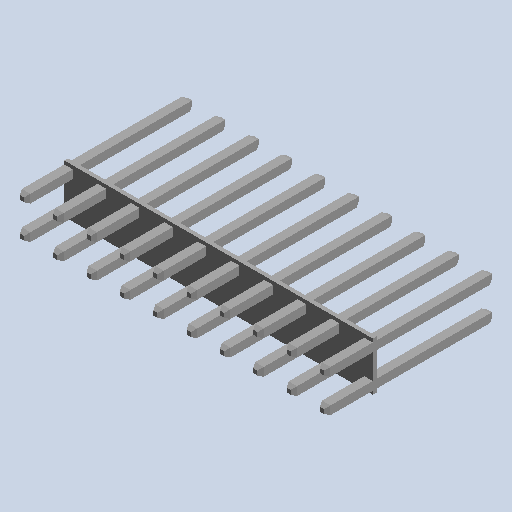
# Autodesk Inventor part: P3TW-10-11-T-D-250-080
Saved by Autodesk Inventor 2024.2 (Build 282272000, 272)
## iProperties
Category: PARTsolutions
Company: SAMTEC
Part Number: P3TW-10-11-T-D-250-080
Material: Generic
Catalog Web Link: www.cadenas.de
Description: TW-TH Pin-TW-TH Series
Vendor: SAMTEC
Document SubType Name: Modeling
Designer: partserver
Manufacturer: SAMTEC
Mass: 0.0621315 g
Surface Area: 5.07361 cm^2
Volume: 0.0621315 cm^3
Density: 1 g/cm^3
Appearance: PSOLRGB-191-191-191
PSOL_IDENT_0: {$CADENAS_DATA\23d-libs\samtec\modelling\tw\parts\tw-th_pin.prj},243 {VTYP=3D},{NB=P3TW-10-11-T-D-25
PSOL_IDENT_1: 0-080},{LINA=P3TW-10-11-T-D-250-080},{NN=TW-TH Pin},{DATE=29.08.2019 09:17:22},{GEOMDATE=10.06.2019
PSOL_IDENT_2: 09:23:15},{VERSION=},{LINEID=10},{WBVAR=PINS,LEADST,PLOPT,ROWOPT,STACKERH,TAILL,POLARIZE},{WBNUMERIC=
PSOL_IDENT_3: STACKERH}  {NB=P3TW-10-11-T-D-250-080},{LINA=P3TW-10-11-T-D-250-080},{KT=DUMMY},{PN=TW-10-11-T-D-250
PSOL_IDENT_4: -080},{SERIES=TW-TH},{PINS=10},{LEADST=11},{LEADSTALG=},{PLOPT=T},{PLOPTALG= '-L','10micro\" (0,25 m
PSOL_IDENT_5: icrom) Gold on contact, Matte Tin on tail','-S','30micro\" (0,76 microm) Gold on contact, Matte Tin
PSOL_IDENT_6: on tail' },{ROWOPT=D},{ROWOPTALG= '5','5:Five Row','6','6:Six Row','D','D:Double Row','Q','Q:Quad Ro
PSOL_IDENT_7: w','S','S:Single row','T','T:Triple Row' },{STACKERH=250},{STACKERHALG=[120:397/5]},{TAILL=080},{TAI
PSOL_IDENT_8: LLALG='000','005','010','015','020','025','030','035','040','045','050','055','060','065','070','075'
PSOL_IDENT_9: ,'080','085','090','095','100','105','110','115','120','125','130','135','140','145'},{ALIGNMENTALG=
PSOL_IDENT_10: x},{POLARIZE=Not Selected},{POLARIZEALG='001','002','003','004','005','006','007','008','009','010','
PSOL_IDENT_11: 011','012','013','014','015','016','017','018','019','020'},{POLARIZEPN=},{KOPTALG= '','Not Selected'
PSOL_IDENT_12: ,'-P','P:Plastic Pick and Place Pad' },{TROPTALG= '','Not Selected','-TR','TR:Tape and Reel' },{IMAT=
PSOL_IDENT_13: Black Liquid Crystal Polymer},{TM=Phosphor Bronze},{PLAT=Au or Sn over 50micro\" (1,27 microm) Ni},{
PSOL_IDENT_14: CR=5.2 A per pin (1 pin powered per row)},{OTEMP=-55°C to +125°C},{ROHSC=Yes},{L=0.7874},{W=0.1574},
PSOL_IDENT_15: {OAL=0.397},{STACKERHMAX=397},{POLMAX='001','002','003','004','005','006','007','008','009','010','0
PSOL_IDENT_16: 11','012','013','014','015','016','017','018','019','020','021','022','023','024','025','026','027','
PSOL_IDENT_17: 028','029','030','031','032','033','034','035','036','037','038','039','040','041','042','043','044'
PSOL_IDENT_18: ,'045','046','047','048','049','050','051','052','053','054','055','056','057','058','059','060','06
PSOL_IDENT_19: 1','062','063','064','065','066','067','068','069','070','071','072','073','074','075','076','077','
PSOL_IDENT_20: 078','079','080','081','082','083','084','085','086','087','088','089','090','091','092','093','094'
PSOL_IDENT_21: ,'095','096','097','098','099','100','101','102','103','104','105','106','107','108','109','110','11
PSOL_IDENT_22: 1','112','113','114','115','116','117','118','119','120','121','122','123','124','125','126','127','
PSOL_IDENT_23: 128','129','130','131','132','133','134','135','136','137','138','139','140','141','142','143','144'
PSOL_IDENT_24: ,'145','146','147','148','149','150','151','152','153','154','155','156','157','158','159','160','16
PSOL_IDENT_25: 1','162','163','164','165','166','167','168','169','170','171','172','173','174','175','176','177','
PSOL_IDENT_26: 178','179','180','181','182','183','184','185','186','187','188','189','190','191','192','193','194'
PSOL_IDENT_27: ,'195','196','197','198','199','200','201','202','203','204','205','206','207','208','209','210','21
PSOL_IDENT_28: 1','212','213','214','215','216','217','218','219','220','221','222','223','224','225','226','227','
PSOL_IDENT_29: 228','229','230','231','232','233','234','235','236','237','238','239','240','241','242','243','244'
PSOL_IDENT_30: ,'245','246','247','248','249','250','251','252','253','254','255','256','257','258','259','260','26
PSOL_IDENT_31: 1','262','263','264','265','266','267','268','269','270','271','272','273','274','275','276','277','
PSOL_IDENT_32: 278','279','280','281','282','283','284','285','286','287','288','289','290','291','292','293','294'
PSOL_IDENT_33: ,'295','296','297','298','299','300'},{TEST2='001','002','003','004','005','006','007','008','009','
PSOL_IDENT_34: 010','011','012','013','014','015','016','017','018','019','020'},{TRUNC=20},{MIN=0.147},{PINSNUM=10
PSOL_IDENT_35: },{POLLR=0},{TAILLMAX=147},{TAILLRANGE='000','005','010','015','020','025','030','035','040','045','
PSOL_IDENT_36: 050','055','060','065','070','075','080','085','090','095','100','105','110','115','120','125','130'
PSOL_IDENT_37: ,'135','140','145','150','155','160','165','170','175','180','185','190','195','200','205','210','21
PSOL_IDENT_38: 5','220','225','230','235','240','245','250','255','260','265','270','275','280','285','290','295','
PSOL_IDENT_39: 300','305','310','315','320','325','330','335','340','345','350','355','360','365','370','375','380'
PSOL_IDENT_40: ,'385','390','395','400','405','410','415','420','425','430','435','440','445','450','455','460','46
PSOL_IDENT_41: 5','470','475','480','485','490','495','500','505','510','515','520','525','530','535','540','545','
PSOL_IDENT_42: 550','555','560','565','570','575','580','585','590','595','600','605','610','615','620','625','630'
PSOL_IDENT_43: ,'635','640','645','650','655','660','665','670','675','680','685','690','695','700','705','710','71
PSOL_IDENT_44: 5','720','725','730','735','740','745','750','755','760','765','770','775','780','785','790','795','
PSOL_IDENT_45: 800','805','810','815','820','825','830','835','840','845','850','855','860','865','870','875','880'
PSOL_IDENT_46: ,'885','890','895','900','905','910','915','920','925','930','935','940','945','950','955','960','96
PSOL_IDENT_47: 5','970','975','980','985','990','995'},{TAILLTRUNC=30},{TAILLNUM=0.08},{ROWNO=2},{POLPLANEPOS=0},{P
PSOL_IDENT_48: OLPINPOS=0},{COLOR=0.75,0.75,0.75,0.00}
NB: P3TW-10-11-T-D-250-080
NN: TW-TH Pin
NT: TW-TH Series
NBSYN: P3$PN.
LINA: P3TW-10-11-T-D-250-080
CATALOG: Samtec
SERIES: TW-TH
PINS: 10
LEADST: 11
PLOPT: -T: Matte Tin Contact and Tail
ROWOPT: D:Double Row
STACKERH: 250
TAILL: 080
POLARIZE: Not Selected
IMAT: Black Liquid Crystal Polymer
TM: Phosphor Bronze
PLAT: Au or Sn over 50micro" (1,27 microm) Ni
CR: 5.2 A per pin (1 pin powered per row)
OTEMP: -55°C to +125°C
ROHSC: Yes
POLMAX: '001','002','003','004','005','006','007','008','009','010','011','012','013','014','015','016','017','018','019','020','021','022','023','024','025','026','027','028','029','030','031','032','033','034','035','036','037','038','039','040','041','042','043','044','045','046','047','048','049','050','051','052','053','054','055','056','057','058','059','060','061','062','063','064','065','066','067','068','069','070','071','072','073','074','075','076','077','078','079','080','081','082','083','084','085','086','087','088','089','090','091','092','093','094','095','096','097','098','099','100','101','102','103','104','105','106','107','108','109','110','111','112','113','114','115','116','117','118','119','120','121','122','123','124','125','126','127','128','129','130','131','132','133','134','135','136','137','138','139','140','141','142','143','144','145','146','147','148','149','150','151','152','153','154','155','156','157','158','159','160','161','162','163','164','165','166','167','168','169','170','171','172','173','174','175','176','177','178','179','180','181','182','183','184','185','186','187','188','189','190','191','192','193','194','195','196','197','198','199','200','201','202','203','204','205','206','207','208','209','210','211','212','213','214','215','216','217','218','219','220','221','222','223','224','225','226','227','228','229','230','231','232','233','234','235','236','237','238','239','240','241','242','243','244','245','246','247','248','249','250','251','252','253','254','255','256','257','258','259','260','261','262','263','264','265','266','267','268','269','270','271','272','273','274','275','276','277','278','279','280','281','282','283','284','285','286','287','288','289','290','291','292','293','294','295','296','297','298','299','300'
TAILLRANGE: '000','005','010','015','020','025','030','035','040','045','050','055','060','065','070','075','080','085','090','095','100','105','110','115','120','125','130','135','140','145','150','155','160','165','170','175','180','185','190','195','200','205','210','215','220','225','230','235','240','245','250','255','260','265','270','275','280','285','290','295','300','305','310','315','320','325','330','335','340','345','350','355','360','365','370','375','380','385','390','395','400','405','410','415','420','425','430','435','440','445','450','455','460','465','470','475','480','485','490','495','500','505','510','515','520','525','530','535','540','545','550','555','560','565','570','575','580','585','590','595','600','605','610','615','620','625','630','635','640','645','650','655','660','665','670','675','680','685','690','695','700','705','710','715','720','725','730','735','740','745','750','755','760','765','770','775','780','785','790','795','800','805','810','815','820','825','830','835','840','845','850','855','860','865','870','875','880','885','890','895','900','905','910','915','920','925','930','935','940','945','950','955','960','965','970','975','980','985','990','995'
SUPPLIER: SAMTEC
ARTICLENO: P3TW-10-11-T-D-250-080
BOMINFO: P3TW-10-11-T-D-250-080
CREATOR: CADENAS GmbH
Title: P3TW-10-11-T-D-250-080
Author: Cadenas PARTsolutions
Comments: TW-TH Series
Autodesk Inventor part; units mm, degrees
sketch "Sketch_2" plane through (9.254, 0, 0) normal (1, 0, 0) x (0, 0, -1)
  line L0 (-1.4605, 0.762) -> (-1.254, 0.762)
  line L1 (-1.254, 0.762) -> (-1.254, -1.778)
  line L2 (-1.254, -1.778) -> (-1.127, -2.032)
  line L3 (-1.127, -2.032) -> (-0.873, -2.032)
  line L4 (-0.873, -2.032) -> (-0.746, -1.778)
  line L5 (-0.746, -1.778) -> (-0.746, 0.762)
  line L6 (-0.746, 0.762) -> (0.746, 0.762)
  line L7 (0.746, 0.762) -> (0.746, -1.778)
  line L8 (0.746, -1.778) -> (0.873, -2.032)
  line L9 (0.873, -2.032) -> (1.127, -2.032)
  line L10 (1.127, -2.032) -> (1.254, -1.778)
  line L11 (1.254, -1.778) -> (1.254, 0.762)
  line L12 (1.254, 0.762) -> (1.4605, 0.762)
  line L13 (1.4605, 0.762) -> (1.4605, 0.9906)
  line L14 (1.4605, 0.9906) -> (1.254, 0.9906)
  line L15 (1.254, 0.9906) -> (1.254, 7.7978)
  line L16 (1.254, 7.7978) -> (1.127, 8.0518)
  line L17 (1.127, 8.0518) -> (0.873, 8.0518)
  line L18 (0.873, 8.0518) -> (0.746, 7.7978)
  line L19 (0.746, 7.7978) -> (0.746, 0.9906)
  line L20 (0.746, 0.9906) -> (-0.746, 0.9906)
  line L21 (-0.746, 0.9906) -> (-0.746, 7.7978)
  line L22 (-0.746, 7.7978) -> (-0.873, 8.0518)
  line L23 (-0.873, 8.0518) -> (-1.127, 8.0518)
  line L24 (-1.127, 8.0518) -> (-1.254, 7.7978)
  line L25 (-1.254, 7.7978) -> (-1.254, 0.9906)
  line L26 (-1.254, 0.9906) -> (-1.4605, 0.9906)
  line L27 (-1.4605, 0.9906) -> (-1.4605, 0.762)
  constraints: 56 end point
extrude "Extrusion1" add sketch "Sketch_2" against normal blind 18.508
sketch "Sketch_1" plane through (0, 0, 0) normal (0, 0, 1) x (1, 0, 0)
  line L0 (-109.4334, 38.1) -> (-109.4334, -38.1)
  line L1 (-109.4334, -38.1) -> (56.7986, -38.1)
  line L2 (56.7986, -38.1) -> (56.7986, 38.1)
  line L3 (56.7986, 38.1) -> (-109.4334, 38.1)
  line L4 (-93.4603, 0.762) -> (-93.2538, 0.762)
  line L5 (-93.2538, 0.762) -> (-93.2538, -1.778)
  line L6 (-93.2538, -1.778) -> (-93.1268, -2.032)
  line L7 (-93.1268, -2.032) -> (-92.8728, -2.032)
  line L8 (-92.8728, -2.032) -> (-92.7458, -1.778)
  line L9 (-92.7458, -1.778) -> (-92.7458, 0.762)
  line L10 (-92.7458, 0.762) -> (-91.2538, 0.762)
  line L11 (-91.2538, 0.762) -> (-91.2538, -1.778)
  line L12 (-91.2538, -1.778) -> (-91.1268, -2.032)
  line L13 (-91.1268, -2.032) -> (-90.8728, -2.032)
  line L14 (-90.8728, -2.032) -> (-90.7458, -1.778)
  line L15 (-90.7458, -1.778) -> (-90.7458, 0.762)
  line L16 (-90.7458, 0.762) -> (-89.2538, 0.762)
  line L17 (-89.2538, 0.762) -> (-89.2538, -1.778)
  line L18 (-89.2538, -1.778) -> (-89.1268, -2.032)
  line L19 (-89.1268, -2.032) -> (-88.8728, -2.032)
  line L20 (-88.8728, -2.032) -> (-88.7458, -1.778)
  line L21 (-88.7458, -1.778) -> (-88.7458, 0.762)
  line L22 (-88.7458, 0.762) -> (-87.2538, 0.762)
  line L23 (-87.2538, 0.762) -> (-87.2538, -1.778)
  line L24 (-87.2538, -1.778) -> (-87.1268, -2.032)
  line L25 (-87.1268, -2.032) -> (-86.8728, -2.032)
  line L26 (-86.8728, -2.032) -> (-86.7458, -1.778)
  line L27 (-86.7458, -1.778) -> (-86.7458, 0.762)
  line L28 (-86.7458, 0.762) -> (-85.2538, 0.762)
  line L29 (-85.2538, 0.762) -> (-85.2538, -1.778)
  line L30 (-85.2538, -1.778) -> (-85.1268, -2.032)
  line L31 (-85.1268, -2.032) -> (-84.8728, -2.032)
  line L32 (-84.8728, -2.032) -> (-84.7458, -1.778)
  line L33 (-84.7458, -1.778) -> (-84.7458, 0.762)
  line L34 (-84.7458, 0.762) -> (-83.2538, 0.762)
  line L35 (-83.2538, 0.762) -> (-83.2538, -1.778)
  line L36 (-83.2538, -1.778) -> (-83.1268, -2.032)
  line L37 (-83.1268, -2.032) -> (-82.8728, -2.032)
  line L38 (-82.8728, -2.032) -> (-82.7458, -1.778)
  line L39 (-82.7458, -1.778) -> (-82.7458, 0.762)
  line L40 (-82.7458, 0.762) -> (-81.2538, 0.762)
  line L41 (-81.2538, 0.762) -> (-81.2538, -1.778)
  line L42 (-81.2538, -1.778) -> (-81.1268, -2.032)
  line L43 (-81.1268, -2.032) -> (-80.8728, -2.032)
  line L44 (-80.8728, -2.032) -> (-80.7458, -1.778)
  line L45 (-80.7458, -1.778) -> (-80.7458, 0.762)
  line L46 (-80.7458, 0.762) -> (-79.2538, 0.762)
  line L47 (-79.2538, 0.762) -> (-79.2538, -1.778)
  line L48 (-79.2538, -1.778) -> (-79.1268, -2.032)
  line L49 (-79.1268, -2.032) -> (-78.8728, -2.032)
  line L50 (-78.8728, -2.032) -> (-78.7458, -1.778)
  line L51 (-78.7458, -1.778) -> (-78.7458, 0.762)
  line L52 (-78.7458, 0.762) -> (-77.2538, 0.762)
  line L53 (-77.2538, 0.762) -> (-77.2538, -1.778)
  line L54 (-77.2538, -1.778) -> (-77.1268, -2.032)
  line L55 (-77.1268, -2.032) -> (-76.8728, -2.032)
  line L56 (-76.8728, -2.032) -> (-76.7458, -1.778)
  line L57 (-76.7458, -1.778) -> (-76.7458, 0.762)
  line L58 (-76.7458, 0.762) -> (-75.2539, 0.762)
  line L59 (-75.2539, 0.762) -> (-75.2539, -1.778)
  line L60 (-75.2539, -1.778) -> (-75.1268, -2.032)
  line L61 (-75.1268, -2.032) -> (-74.8728, -2.032)
  line L62 (-74.8728, -2.032) -> (-74.7459, -1.778)
  line L63 (-74.7459, -1.778) -> (-74.7459, 0.762)
  line L64 (-74.7459, 0.762) -> (-73.2539, 0.762)
  line L65 (-73.2539, 0.762) -> (-73.2539, -1.778)
  line L66 (-73.2539, -1.778) -> (-73.1269, -2.032)
  line L67 (-73.1269, -2.032) -> (-72.8729, -2.032)
  line L68 (-72.8729, -2.032) -> (-72.7459, -1.778)
  line L69 (-72.7459, -1.778) -> (-72.7459, 0.762)
  line L70 (-72.7459, 0.762) -> (-71.2539, 0.762)
  line L71 (-71.2539, 0.762) -> (-71.2539, -1.778)
  line L72 (-71.2539, -1.778) -> (-71.1269, -2.032)
  line L73 (-71.1269, -2.032) -> (-70.8729, -2.032)
  line L74 (-70.8729, -2.032) -> (-70.7459, -1.778)
  line L75 (-70.7459, -1.778) -> (-70.7459, 0.762)
  line L76 (-70.7459, 0.762) -> (-69.2539, 0.762)
  line L77 (-69.2539, 0.762) -> (-69.2539, -1.778)
  line L78 (-69.2539, -1.778) -> (-69.1269, -2.032)
  line L79 (-69.1269, -2.032) -> (-68.8729, -2.032)
  line L80 (-68.8729, -2.032) -> (-68.7459, -1.778)
  line L81 (-68.7459, -1.778) -> (-68.7459, 0.762)
  line L82 (-68.7459, 0.762) -> (-67.2539, 0.762)
  line L83 (-67.2539, 0.762) -> (-67.2539, -1.778)
  line L84 (-67.2539, -1.778) -> (-67.1269, -2.032)
  line L85 (-67.1269, -2.032) -> (-66.8729, -2.032)
  line L86 (-66.8729, -2.032) -> (-66.7459, -1.778)
  line L87 (-66.7459, -1.778) -> (-66.7459, 0.762)
  line L88 (-66.7459, 0.762) -> (-65.2539, 0.762)
  line L89 (-65.2539, 0.762) -> (-65.2539, -1.778)
  line L90 (-65.2539, -1.778) -> (-65.1269, -2.032)
  line L91 (-65.1269, -2.032) -> (-64.8729, -2.032)
  line L92 (-64.8729, -2.032) -> (-64.7459, -1.778)
  line L93 (-64.7459, -1.778) -> (-64.7459, 0.762)
  line L94 (-64.7459, 0.762) -> (-63.2539, 0.762)
  line L95 (-63.2539, 0.762) -> (-63.2539, -1.778)
  line L96 (-63.2539, -1.778) -> (-63.1269, -2.032)
  line L97 (-63.1269, -2.032) -> (-62.8729, -2.032)
  line L98 (-62.8729, -2.032) -> (-62.7459, -1.778)
  line L99 (-62.7459, -1.778) -> (-62.7459, 0.762)
  line L100 (-62.7459, 0.762) -> (-61.2539, 0.762)
  line L101 (-61.2539, 0.762) -> (-61.2539, -1.778)
  line L102 (-61.2539, -1.778) -> (-61.1269, -2.032)
  line L103 (-61.1269, -2.032) -> (-60.8729, -2.032)
  line L104 (-60.8729, -2.032) -> (-60.7459, -1.778)
  line L105 (-60.7459, -1.778) -> (-60.7459, 0.762)
  line L106 (-60.7459, 0.762) -> (-59.2539, 0.762)
  line L107 (-59.2539, 0.762) -> (-59.2539, -1.778)
  line L108 (-59.2539, -1.778) -> (-59.1269, -2.032)
  line L109 (-59.1269, -2.032) -> (-58.8729, -2.032)
  line L110 (-58.8729, -2.032) -> (-58.7459, -1.778)
  line L111 (-58.7459, -1.778) -> (-58.7459, 0.762)
  line L112 (-58.7459, 0.762) -> (-57.2539, 0.762)
  line L113 (-57.2539, 0.762) -> (-57.2539, -1.778)
  line L114 (-57.2539, -1.778) -> (-57.1269, -2.032)
  line L115 (-57.1269, -2.032) -> (-56.8729, -2.032)
  line L116 (-56.8729, -2.032) -> (-56.7459, -1.778)
  line L117 (-56.7459, -1.778) -> (-56.7459, 0.762)
  line L118 (-56.7459, 0.762) -> (-55.2539, 0.762)
  line L119 (-55.2539, 0.762) -> (-55.2539, -1.778)
  line L120 (-55.2539, -1.778) -> (-55.1269, -2.032)
  line L121 (-55.1269, -2.032) -> (-54.8729, -2.032)
  line L122 (-54.8729, -2.032) -> (-54.7459, -1.778)
  line L123 (-54.7459, -1.778) -> (-54.7459, 0.762)
  line L124 (-54.7459, 0.762) -> (-53.2539, 0.762)
  line L125 (-53.2539, 0.762) -> (-53.2539, -1.778)
  line L126 (-53.2539, -1.778) -> (-53.1269, -2.032)
  line L127 (-53.1269, -2.032) -> (-52.8729, -2.032)
  line L128 (-52.8729, -2.032) -> (-52.7459, -1.778)
  line L129 (-52.7459, -1.778) -> (-52.7459, 0.762)
  line L130 (-52.7459, 0.762) -> (-51.2539, 0.762)
  line L131 (-51.2539, 0.762) -> (-51.2539, -1.778)
  line L132 (-51.2539, -1.778) -> (-51.1269, -2.032)
  line L133 (-51.1269, -2.032) -> (-50.8729, -2.032)
  line L134 (-50.8729, -2.032) -> (-50.7459, -1.778)
  line L135 (-50.7459, -1.778) -> (-50.7459, 0.762)
  line L136 (-50.7459, 0.762) -> (-49.2539, 0.762)
  line L137 (-49.2539, 0.762) -> (-49.2539, -1.778)
  line L138 (-49.2539, -1.778) -> (-49.1269, -2.032)
  line L139 (-49.1269, -2.032) -> (-48.8729, -2.032)
  line L140 (-48.8729, -2.032) -> (-48.7459, -1.778)
  line L141 (-48.7459, -1.778) -> (-48.7459, 0.762)
  line L142 (-48.7459, 0.762) -> (-47.2539, 0.762)
  line L143 (-47.2539, 0.762) -> (-47.2539, -1.778)
  line L144 (-47.2539, -1.778) -> (-47.1269, -2.032)
  line L145 (-47.1269, -2.032) -> (-46.8729, -2.032)
  line L146 (-46.8729, -2.032) -> (-46.7459, -1.778)
  line L147 (-46.7459, -1.778) -> (-46.7459, 0.762)
  line L148 (-46.7459, 0.762) -> (-45.2539, 0.762)
  line L149 (-45.2539, 0.762) -> (-45.2539, -1.778)
  line L150 (-45.2539, -1.778) -> (-45.1269, -2.032)
  line L151 (-45.1269, -2.032) -> (-44.8729, -2.032)
  line L152 (-44.8729, -2.032) -> (-44.7459, -1.778)
  line L153 (-44.7459, -1.778) -> (-44.7459, 0.762)
  line L154 (-44.7459, 0.762) -> (-43.2539, 0.762)
  line L155 (-43.2539, 0.762) -> (-43.2539, -1.778)
  line L156 (-43.2539, -1.778) -> (-43.1269, -2.032)
  line L157 (-43.1269, -2.032) -> (-42.8729, -2.032)
  line L158 (-42.8729, -2.032) -> (-42.7459, -1.778)
  line L159 (-42.7459, -1.778) -> (-42.7459, 0.762)
  line L160 (-42.7459, 0.762) -> (-41.2539, 0.762)
  line L161 (-41.2539, 0.762) -> (-41.2539, -1.778)
  line L162 (-41.2539, -1.778) -> (-41.1269, -2.032)
  line L163 (-41.1269, -2.032) -> (-40.8729, -2.032)
  line L164 (-40.8729, -2.032) -> (-40.7459, -1.778)
  line L165 (-40.7459, -1.778) -> (-40.7459, 0.762)
  line L166 (-40.7459, 0.762) -> (-39.2539, 0.762)
  line L167 (-39.2539, 0.762) -> (-39.2539, -1.778)
  line L168 (-39.2539, -1.778) -> (-39.1269, -2.032)
  line L169 (-39.1269, -2.032) -> (-38.8729, -2.032)
  line L170 (-38.8729, -2.032) -> (-38.7459, -1.778)
  line L171 (-38.7459, -1.778) -> (-38.7459, 0.762)
  line L172 (-38.7459, 0.762) -> (-37.2539, 0.762)
  line L173 (-37.2539, 0.762) -> (-37.2539, -1.778)
  line L174 (-37.2539, -1.778) -> (-37.1269, -2.032)
  line L175 (-37.1269, -2.032) -> (-36.8729, -2.032)
  line L176 (-36.8729, -2.032) -> (-36.7459, -1.778)
  line L177 (-36.7459, -1.778) -> (-36.7459, 0.762)
  line L178 (-36.7459, 0.762) -> (-35.2539, 0.762)
  line L179 (-35.2539, 0.762) -> (-35.2539, -1.778)
  line L180 (-35.2539, -1.778) -> (-35.1269, -2.032)
  line L181 (-35.1269, -2.032) -> (-34.8729, -2.032)
  line L182 (-34.8729, -2.032) -> (-34.7459, -1.778)
  line L183 (-34.7459, -1.778) -> (-34.7459, 0.762)
  line L184 (-34.7459, 0.762) -> (-33.2539, 0.762)
  line L185 (-33.2539, 0.762) -> (-33.2539, -1.778)
  line L186 (-33.2539, -1.778) -> (-33.1269, -2.032)
  line L187 (-33.1269, -2.032) -> (-32.8729, -2.032)
  line L188 (-32.8729, -2.032) -> (-32.7459, -1.778)
  line L189 (-32.7459, -1.778) -> (-32.7459, 0.762)
  line L190 (-32.7459, 0.762) -> (-31.2539, 0.762)
  line L191 (-31.2539, 0.762) -> (-31.2539, -1.778)
  line L192 (-31.2539, -1.778) -> (-31.1269, -2.032)
  line L193 (-31.1269, -2.032) -> (-30.8729, -2.032)
  line L194 (-30.8729, -2.032) -> (-30.7459, -1.778)
  line L195 (-30.7459, -1.778) -> (-30.7459, 0.762)
  line L196 (-30.7459, 0.762) -> (-29.2539, 0.762)
  line L197 (-29.2539, 0.762) -> (-29.2539, -1.778)
  line L198 (-29.2539, -1.778) -> (-29.1269, -2.032)
  line L199 (-29.1269, -2.032) -> (-28.8729, -2.032)
  line L200 (-28.8729, -2.032) -> (-28.7459, -1.778)
  line L201 (-28.7459, -1.778) -> (-28.7459, 0.762)
  line L202 (-28.7459, 0.762) -> (-27.2539, 0.762)
  line L203 (-27.2539, 0.762) -> (-27.2539, -1.778)
  line L204 (-27.2539, -1.778) -> (-27.1269, -2.032)
  line L205 (-27.1269, -2.032) -> (-26.8729, -2.032)
  line L206 (-26.8729, -2.032) -> (-26.7459, -1.778)
  line L207 (-26.7459, -1.778) -> (-26.7459, 0.762)
  line L208 (-26.7459, 0.762) -> (-25.2539, 0.762)
  line L209 (-25.2539, 0.762) -> (-25.2539, -1.778)
  line L210 (-25.2539, -1.778) -> (-25.127, -2.032)
  line L211 (-25.127, -2.032) -> (-24.8729, -2.032)
  line L212 (-24.8729, -2.032) -> (-24.746, -1.778)
  line L213 (-24.746, -1.778) -> (-24.746, 0.762)
  line L214 (-24.746, 0.762) -> (-23.254, 0.762)
  line L215 (-23.254, 0.762) -> (-23.254, -1.778)
  line L216 (-23.254, -1.778) -> (-23.127, -2.032)
  line L217 (-23.127, -2.032) -> (-22.873, -2.032)
  line L218 (-22.873, -2.032) -> (-22.746, -1.778)
  line L219 (-22.746, -1.778) -> (-22.746, 0.762)
  line L220 (-22.746, 0.762) -> (-21.254, 0.762)
  line L221 (-21.254, 0.762) -> (-21.254, -1.778)
  line L222 (-21.254, -1.778) -> (-21.127, -2.032)
  line L223 (-21.127, -2.032) -> (-20.873, -2.032)
  line L224 (-20.873, -2.032) -> (-20.746, -1.778)
  line L225 (-20.746, -1.778) -> (-20.746, 0.762)
  line L226 (-20.746, 0.762) -> (-19.254, 0.762)
  line L227 (-19.254, 0.762) -> (-19.254, -1.778)
  line L228 (-19.254, -1.778) -> (-19.127, -2.032)
  line L229 (-19.127, -2.032) -> (-18.873, -2.032)
  line L230 (-18.873, -2.032) -> (-18.746, -1.778)
  line L231 (-18.746, -1.778) -> (-18.746, 0.762)
  line L232 (-18.746, 0.762) -> (-17.254, 0.762)
  line L233 (-17.254, 0.762) -> (-17.254, -1.778)
  line L234 (-17.254, -1.778) -> (-17.127, -2.032)
  line L235 (-17.127, -2.032) -> (-16.873, -2.032)
  line L236 (-16.873, -2.032) -> (-16.746, -1.778)
  line L237 (-16.746, -1.778) -> (-16.746, 0.762)
  line L238 (-16.746, 0.762) -> (-15.254, 0.762)
  line L239 (-15.254, 0.762) -> (-15.254, -1.778)
  line L240 (-15.254, -1.778) -> (-15.127, -2.032)
  line L241 (-15.127, -2.032) -> (-14.873, -2.032)
  line L242 (-14.873, -2.032) -> (-14.746, -1.778)
  line L243 (-14.746, -1.778) -> (-14.746, 0.762)
  line L244 (-14.746, 0.762) -> (-13.254, 0.762)
  line L245 (-13.254, 0.762) -> (-13.254, -1.778)
  line L246 (-13.254, -1.778) -> (-13.127, -2.032)
  line L247 (-13.127, -2.032) -> (-12.873, -2.032)
  line L248 (-12.873, -2.032) -> (-12.746, -1.778)
  line L249 (-12.746, -1.778) -> (-12.746, 0.762)
  line L250 (-12.746, 0.762) -> (-11.254, 0.762)
  line L251 (-11.254, 0.762) -> (-11.254, -1.778)
  line L252 (-11.254, -1.778) -> (-11.127, -2.032)
  line L253 (-11.127, -2.032) -> (-10.873, -2.032)
  line L254 (-10.873, -2.032) -> (-10.746, -1.778)
  line L255 (-10.746, -1.778) -> (-10.746, 0.762)
  line L256 (-10.746, 0.762) -> (-9.254, 0.762)
  line L257 (-9.254, 0.762) -> (-9.254, -1.778)
  line L258 (-9.254, -1.778) -> (-9.127, -2.032)
  line L259 (-9.127, -2.032) -> (-8.873, -2.032)
  line L260 (-8.873, -2.032) -> (-8.746, -1.778)
  line L261 (-8.746, -1.778) -> (-8.746, 0.762)
  line L262 (-8.746, 0.762) -> (-7.254, 0.762)
  line L263 (-7.254, 0.762) -> (-7.254, -1.778)
  line L264 (-7.254, -1.778) -> (-7.127, -2.032)
  line L265 (-7.127, -2.032) -> (-6.873, -2.032)
  line L266 (-6.873, -2.032) -> (-6.746, -1.778)
  line L267 (-6.746, -1.778) -> (-6.746, 0.762)
  line L268 (-6.746, 0.762) -> (-5.254, 0.762)
  line L269 (-5.254, 0.762) -> (-5.254, -1.778)
  line L270 (-5.254, -1.778) -> (-5.127, -2.032)
  line L271 (-5.127, -2.032) -> (-4.873, -2.032)
  line L272 (-4.873, -2.032) -> (-4.746, -1.778)
  line L273 (-4.746, -1.778) -> (-4.746, 0.762)
  line L274 (-4.746, 0.762) -> (-3.254, 0.762)
  line L275 (-3.254, 0.762) -> (-3.254, -1.778)
  line L276 (-3.254, -1.778) -> (-3.127, -2.032)
  line L277 (-3.127, -2.032) -> (-2.873, -2.032)
  line L278 (-2.873, -2.032) -> (-2.746, -1.778)
  line L279 (-2.746, -1.778) -> (-2.746, 0.762)
  line L280 (-2.746, 0.762) -> (-1.254, 0.762)
  line L281 (-1.254, 0.762) -> (-1.254, -1.778)
  line L282 (-1.254, -1.778) -> (-1.127, -2.032)
  line L283 (-1.127, -2.032) -> (-0.873, -2.032)
  line L284 (-0.873, -2.032) -> (-0.746, -1.778)
  line L285 (-0.746, -1.778) -> (-0.746, 0.762)
  line L286 (-0.746, 0.762) -> (0.746, 0.762)
  line L287 (0.746, 0.762) -> (0.746, -1.778)
  line L288 (0.746, -1.778) -> (0.873, -2.032)
  line L289 (0.873, -2.032) -> (1.127, -2.032)
  line L290 (1.127, -2.032) -> (1.254, -1.778)
  line L291 (1.254, -1.778) -> (1.254, 0.762)
  line L292 (1.254, 0.762) -> (2.746, 0.762)
  line L293 (2.746, 0.762) -> (2.746, -1.778)
  line L294 (2.746, -1.778) -> (2.873, -2.032)
  line L295 (2.873, -2.032) -> (3.127, -2.032)
  line L296 (3.127, -2.032) -> (3.254, -1.778)
  line L297 (3.254, -1.778) -> (3.254, 0.762)
  line L298 (3.254, 0.762) -> (4.746, 0.762)
  line L299 (4.746, 0.762) -> (4.746, -1.778)
  line L300 (4.746, -1.778) -> (4.873, -2.032)
  line L301 (4.873, -2.032) -> (5.127, -2.032)
  line L302 (5.127, -2.032) -> (5.254, -1.778)
  line L303 (5.254, -1.778) -> (5.254, 0.762)
  line L304 (5.254, 0.762) -> (6.746, 0.762)
  line L305 (6.746, 0.762) -> (6.746, -1.778)
  line L306 (6.746, -1.778) -> (6.873, -2.032)
  line L307 (6.873, -2.032) -> (7.127, -2.032)
  line L308 (7.127, -2.032) -> (7.254, -1.778)
  line L309 (7.254, -1.778) -> (7.254, 0.762)
  line L310 (7.254, 0.762) -> (8.746, 0.762)
  line L311 (8.746, 0.762) -> (8.746, -1.778)
  line L312 (8.746, -1.778) -> (8.873, -2.032)
  line L313 (8.873, -2.032) -> (9.127, -2.032)
  line L314 (9.127, -2.032) -> (9.254, -1.778)
  line L315 (9.254, -1.778) -> (9.254, 0.762)
  line L316 (9.254, 0.762) -> (9.4605, 0.762)
  line L317 (9.4605, 0.762) -> (9.4605, 0.9906)
  line L318 (9.4605, 0.9906) -> (9.254, 0.9906)
  line L319 (9.254, 0.9906) -> (9.254, 7.7978)
  line L320 (9.254, 7.7978) -> (9.127, 8.0518)
  line L321 (9.127, 8.0518) -> (8.873, 8.0518)
  line L322 (8.873, 8.0518) -> (8.746, 7.7978)
  line L323 (8.746, 7.7978) -> (8.746, 0.9906)
  line L324 (8.746, 0.9906) -> (7.254, 0.9906)
  line L325 (7.254, 0.9906) -> (7.254, 7.7978)
  line L326 (7.254, 7.7978) -> (7.127, 8.0518)
  line L327 (7.127, 8.0518) -> (6.873, 8.0518)
  line L328 (6.873, 8.0518) -> (6.746, 7.7978)
  line L329 (6.746, 7.7978) -> (6.746, 0.9906)
  line L330 (6.746, 0.9906) -> (5.254, 0.9906)
  line L331 (5.254, 0.9906) -> (5.254, 7.7978)
  line L332 (5.254, 7.7978) -> (5.127, 8.0518)
  line L333 (5.127, 8.0518) -> (4.873, 8.0518)
  line L334 (4.873, 8.0518) -> (4.746, 7.7978)
  line L335 (4.746, 7.7978) -> (4.746, 0.9906)
  line L336 (4.746, 0.9906) -> (3.254, 0.9906)
  line L337 (3.254, 0.9906) -> (3.254, 7.7978)
  line L338 (3.254, 7.7978) -> (3.127, 8.0518)
  line L339 (3.127, 8.0518) -> (2.873, 8.0518)
  line L340 (2.873, 8.0518) -> (2.746, 7.7978)
  line L341 (2.746, 7.7978) -> (2.746, 0.9906)
  line L342 (2.746, 0.9906) -> (1.254, 0.9906)
  line L343 (1.254, 0.9906) -> (1.254, 7.7978)
  line L344 (1.254, 7.7978) -> (1.127, 8.0518)
  line L345 (1.127, 8.0518) -> (0.873, 8.0518)
  line L346 (0.873, 8.0518) -> (0.746, 7.7978)
  line L347 (0.746, 7.7978) -> (0.746, 0.9906)
  line L348 (0.746, 0.9906) -> (-0.746, 0.9906)
  line L349 (-0.746, 0.9906) -> (-0.746, 7.7978)
  line L350 (-0.746, 7.7978) -> (-0.873, 8.0518)
  line L351 (-0.873, 8.0518) -> (-1.127, 8.0518)
  line L352 (-1.127, 8.0518) -> (-1.254, 7.7978)
  line L353 (-1.254, 7.7978) -> (-1.254, 0.9906)
  line L354 (-1.254, 0.9906) -> (-2.746, 0.9906)
  line L355 (-2.746, 0.9906) -> (-2.746, 7.7978)
  line L356 (-2.746, 7.7978) -> (-2.873, 8.0518)
  line L357 (-2.873, 8.0518) -> (-3.127, 8.0518)
  line L358 (-3.127, 8.0518) -> (-3.254, 7.7978)
  line L359 (-3.254, 7.7978) -> (-3.254, 0.9906)
  line L360 (-3.254, 0.9906) -> (-4.746, 0.9906)
  line L361 (-4.746, 0.9906) -> (-4.746, 7.7978)
  line L362 (-4.746, 7.7978) -> (-4.873, 8.0518)
  line L363 (-4.873, 8.0518) -> (-5.127, 8.0518)
  line L364 (-5.127, 8.0518) -> (-5.254, 7.7978)
  line L365 (-5.254, 7.7978) -> (-5.254, 0.9906)
  line L366 (-5.254, 0.9906) -> (-6.746, 0.9906)
  line L367 (-6.746, 0.9906) -> (-6.746, 7.7978)
  line L368 (-6.746, 7.7978) -> (-6.873, 8.0518)
  line L369 (-6.873, 8.0518) -> (-7.127, 8.0518)
  line L370 (-7.127, 8.0518) -> (-7.254, 7.7978)
  line L371 (-7.254, 7.7978) -> (-7.254, 0.9906)
  line L372 (-7.254, 0.9906) -> (-8.746, 0.9906)
  line L373 (-8.746, 0.9906) -> (-8.746, 7.7978)
  line L374 (-8.746, 7.7978) -> (-8.873, 8.0518)
  line L375 (-8.873, 8.0518) -> (-9.127, 8.0518)
  line L376 (-9.127, 8.0518) -> (-9.254, 7.7978)
  line L377 (-9.254, 7.7978) -> (-9.254, 0.9906)
  line L378 (-9.254, 0.9906) -> (-10.746, 0.9906)
  line L379 (-10.746, 0.9906) -> (-10.746, 7.7978)
  line L380 (-10.746, 7.7978) -> (-10.873, 8.0518)
  line L381 (-10.873, 8.0518) -> (-11.127, 8.0518)
  line L382 (-11.127, 8.0518) -> (-11.254, 7.7978)
  line L383 (-11.254, 7.7978) -> (-11.254, 0.9906)
  line L384 (-11.254, 0.9906) -> (-12.746, 0.9906)
  line L385 (-12.746, 0.9906) -> (-12.746, 7.7978)
  line L386 (-12.746, 7.7978) -> (-12.873, 8.0518)
  line L387 (-12.873, 8.0518) -> (-13.127, 8.0518)
  line L388 (-13.127, 8.0518) -> (-13.254, 7.7978)
  line L389 (-13.254, 7.7978) -> (-13.254, 0.9906)
  line L390 (-13.254, 0.9906) -> (-14.746, 0.9906)
  line L391 (-14.746, 0.9906) -> (-14.746, 7.7978)
  line L392 (-14.746, 7.7978) -> (-14.873, 8.0518)
  line L393 (-14.873, 8.0518) -> (-15.127, 8.0518)
  line L394 (-15.127, 8.0518) -> (-15.254, 7.7978)
  line L395 (-15.254, 7.7978) -> (-15.254, 0.9906)
  line L396 (-15.254, 0.9906) -> (-16.746, 0.9906)
  line L397 (-16.746, 0.9906) -> (-16.746, 7.7978)
  line L398 (-16.746, 7.7978) -> (-16.873, 8.0518)
  line L399 (-16.873, 8.0518) -> (-17.127, 8.0518)
  line L400 (-17.127, 8.0518) -> (-17.254, 7.7978)
  line L401 (-17.254, 7.7978) -> (-17.254, 0.9906)
  line L402 (-17.254, 0.9906) -> (-18.746, 0.9906)
  line L403 (-18.746, 0.9906) -> (-18.746, 7.7978)
  line L404 (-18.746, 7.7978) -> (-18.873, 8.0518)
  line L405 (-18.873, 8.0518) -> (-19.127, 8.0518)
  line L406 (-19.127, 8.0518) -> (-19.254, 7.7978)
  line L407 (-19.254, 7.7978) -> (-19.254, 0.9906)
  line L408 (-19.254, 0.9906) -> (-20.746, 0.9906)
  line L409 (-20.746, 0.9906) -> (-20.746, 7.7978)
  line L410 (-20.746, 7.7978) -> (-20.873, 8.0518)
  line L411 (-20.873, 8.0518) -> (-21.127, 8.0518)
  line L412 (-21.127, 8.0518) -> (-21.254, 7.7978)
  line L413 (-21.254, 7.7978) -> (-21.254, 0.9906)
  line L414 (-21.254, 0.9906) -> (-22.746, 0.9906)
  line L415 (-22.746, 0.9906) -> (-22.746, 7.7978)
  line L416 (-22.746, 7.7978) -> (-22.873, 8.0518)
  line L417 (-22.873, 8.0518) -> (-23.127, 8.0518)
  line L418 (-23.127, 8.0518) -> (-23.254, 7.7978)
  line L419 (-23.254, 7.7978) -> (-23.254, 0.9906)
  line L420 (-23.254, 0.9906) -> (-24.746, 0.9906)
  line L421 (-24.746, 0.9906) -> (-24.746, 7.7978)
  line L422 (-24.746, 7.7978) -> (-24.8729, 8.0518)
  line L423 (-24.8729, 8.0518) -> (-25.127, 8.0518)
  line L424 (-25.127, 8.0518) -> (-25.2539, 7.7978)
  line L425 (-25.2539, 7.7978) -> (-25.2539, 0.9906)
  line L426 (-25.2539, 0.9906) -> (-26.7459, 0.9906)
  line L427 (-26.7459, 0.9906) -> (-26.7459, 7.7978)
  line L428 (-26.7459, 7.7978) -> (-26.8729, 8.0518)
  line L429 (-26.8729, 8.0518) -> (-27.1269, 8.0518)
  line L430 (-27.1269, 8.0518) -> (-27.2539, 7.7978)
  line L431 (-27.2539, 7.7978) -> (-27.2539, 0.9906)
  line L432 (-27.2539, 0.9906) -> (-28.7459, 0.9906)
  line L433 (-28.7459, 0.9906) -> (-28.7459, 7.7978)
  line L434 (-28.7459, 7.7978) -> (-28.8729, 8.0518)
  line L435 (-28.8729, 8.0518) -> (-29.1269, 8.0518)
  line L436 (-29.1269, 8.0518) -> (-29.2539, 7.7978)
  line L437 (-29.2539, 7.7978) -> (-29.2539, 0.9906)
  line L438 (-29.2539, 0.9906) -> (-30.7459, 0.9906)
  line L439 (-30.7459, 0.9906) -> (-30.7459, 7.7978)
  line L440 (-30.7459, 7.7978) -> (-30.8729, 8.0518)
  line L441 (-30.8729, 8.0518) -> (-31.1269, 8.0518)
  line L442 (-31.1269, 8.0518) -> (-31.2539, 7.7978)
  line L443 (-31.2539, 7.7978) -> (-31.2539, 0.9906)
  line L444 (-31.2539, 0.9906) -> (-32.7459, 0.9906)
  line L445 (-32.7459, 0.9906) -> (-32.7459, 7.7978)
  line L446 (-32.7459, 7.7978) -> (-32.8729, 8.0518)
  line L447 (-32.8729, 8.0518) -> (-33.1269, 8.0518)
  line L448 (-33.1269, 8.0518) -> (-33.2539, 7.7978)
  line L449 (-33.2539, 7.7978) -> (-33.2539, 0.9906)
  line L450 (-33.2539, 0.9906) -> (-34.7459, 0.9906)
  line L451 (-34.7459, 0.9906) -> (-34.7459, 7.7978)
  line L452 (-34.7459, 7.7978) -> (-34.8729, 8.0518)
  line L453 (-34.8729, 8.0518) -> (-35.1269, 8.0518)
  line L454 (-35.1269, 8.0518) -> (-35.2539, 7.7978)
  line L455 (-35.2539, 7.7978) -> (-35.2539, 0.9906)
  line L456 (-35.2539, 0.9906) -> (-36.7459, 0.9906)
  line L457 (-36.7459, 0.9906) -> (-36.7459, 7.7978)
  line L458 (-36.7459, 7.7978) -> (-36.8729, 8.0518)
  line L459 (-36.8729, 8.0518) -> (-37.1269, 8.0518)
  line L460 (-37.1269, 8.0518) -> (-37.2539, 7.7978)
  line L461 (-37.2539, 7.7978) -> (-37.2539, 0.9906)
  line L462 (-37.2539, 0.9906) -> (-38.7459, 0.9906)
  line L463 (-38.7459, 0.9906) -> (-38.7459, 7.7978)
  line L464 (-38.7459, 7.7978) -> (-38.8729, 8.0518)
  line L465 (-38.8729, 8.0518) -> (-39.1269, 8.0518)
  line L466 (-39.1269, 8.0518) -> (-39.2539, 7.7978)
  line L467 (-39.2539, 7.7978) -> (-39.2539, 0.9906)
  line L468 (-39.2539, 0.9906) -> (-40.7459, 0.9906)
  line L469 (-40.7459, 0.9906) -> (-40.7459, 7.7978)
  line L470 (-40.7459, 7.7978) -> (-40.8729, 8.0518)
  line L471 (-40.8729, 8.0518) -> (-41.1269, 8.0518)
  line L472 (-41.1269, 8.0518) -> (-41.2539, 7.7978)
  line L473 (-41.2539, 7.7978) -> (-41.2539, 0.9906)
  line L474 (-41.2539, 0.9906) -> (-42.7459, 0.9906)
  line L475 (-42.7459, 0.9906) -> (-42.7459, 7.7978)
  line L476 (-42.7459, 7.7978) -> (-42.8729, 8.0518)
  line L477 (-42.8729, 8.0518) -> (-43.1269, 8.0518)
  line L478 (-43.1269, 8.0518) -> (-43.2539, 7.7978)
  line L479 (-43.2539, 7.7978) -> (-43.2539, 0.9906)
  line L480 (-43.2539, 0.9906) -> (-44.7459, 0.9906)
  line L481 (-44.7459, 0.9906) -> (-44.7459, 7.7978)
  line L482 (-44.7459, 7.7978) -> (-44.8729, 8.0518)
  line L483 (-44.8729, 8.0518) -> (-45.1269, 8.0518)
  line L484 (-45.1269, 8.0518) -> (-45.2539, 7.7978)
  line L485 (-45.2539, 7.7978) -> (-45.2539, 0.9906)
  line L486 (-45.2539, 0.9906) -> (-46.7459, 0.9906)
  line L487 (-46.7459, 0.9906) -> (-46.7459, 7.7978)
  line L488 (-46.7459, 7.7978) -> (-46.8729, 8.0518)
  line L489 (-46.8729, 8.0518) -> (-47.1269, 8.0518)
  line L490 (-47.1269, 8.0518) -> (-47.2539, 7.7978)
  line L491 (-47.2539, 7.7978) -> (-47.2539, 0.9906)
  line L492 (-47.2539, 0.9906) -> (-48.7459, 0.9906)
  line L493 (-48.7459, 0.9906) -> (-48.7459, 7.7978)
  line L494 (-48.7459, 7.7978) -> (-48.8729, 8.0518)
  line L495 (-48.8729, 8.0518) -> (-49.1269, 8.0518)
  line L496 (-49.1269, 8.0518) -> (-49.2539, 7.7978)
  line L497 (-49.2539, 7.7978) -> (-49.2539, 0.9906)
  line L498 (-49.2539, 0.9906) -> (-50.7459, 0.9906)
  line L499 (-50.7459, 0.9906) -> (-50.7459, 7.7978)
  line L500 (-50.7459, 7.7978) -> (-50.8729, 8.0518)
  line L501 (-50.8729, 8.0518) -> (-51.1269, 8.0518)
  line L502 (-51.1269, 8.0518) -> (-51.2539, 7.7978)
  line L503 (-51.2539, 7.7978) -> (-51.2539, 0.9906)
  line L504 (-51.2539, 0.9906) -> (-52.7459, 0.9906)
  line L505 (-52.7459, 0.9906) -> (-52.7459, 7.7978)
  line L506 (-52.7459, 7.7978) -> (-52.8729, 8.0518)
  line L507 (-52.8729, 8.0518) -> (-53.1269, 8.0518)
  line L508 (-53.1269, 8.0518) -> (-53.2539, 7.7978)
  line L509 (-53.2539, 7.7978) -> (-53.2539, 0.9906)
  line L510 (-53.2539, 0.9906) -> (-54.7459, 0.9906)
  line L511 (-54.7459, 0.9906) -> (-54.7459, 7.7978)
  line L512 (-54.7459, 7.7978) -> (-54.8729, 8.0518)
  line L513 (-54.8729, 8.0518) -> (-55.1269, 8.0518)
  line L514 (-55.1269, 8.0518) -> (-55.2539, 7.7978)
  line L515 (-55.2539, 7.7978) -> (-55.2539, 0.9906)
  line L516 (-55.2539, 0.9906) -> (-56.7459, 0.9906)
  line L517 (-56.7459, 0.9906) -> (-56.7459, 7.7978)
  line L518 (-56.7459, 7.7978) -> (-56.8729, 8.0518)
  line L519 (-56.8729, 8.0518) -> (-57.1269, 8.0518)
  line L520 (-57.1269, 8.0518) -> (-57.2539, 7.7978)
  line L521 (-57.2539, 7.7978) -> (-57.2539, 0.9906)
  line L522 (-57.2539, 0.9906) -> (-58.7459, 0.9906)
  line L523 (-58.7459, 0.9906) -> (-58.7459, 7.7978)
  line L524 (-58.7459, 7.7978) -> (-58.8729, 8.0518)
  line L525 (-58.8729, 8.0518) -> (-59.1269, 8.0518)
  line L526 (-59.1269, 8.0518) -> (-59.2539, 7.7978)
  line L527 (-59.2539, 7.7978) -> (-59.2539, 0.9906)
  line L528 (-59.2539, 0.9906) -> (-60.7459, 0.9906)
  line L529 (-60.7459, 0.9906) -> (-60.7459, 7.7978)
  line L530 (-60.7459, 7.7978) -> (-60.8729, 8.0518)
  line L531 (-60.8729, 8.0518) -> (-61.1269, 8.0518)
  line L532 (-61.1269, 8.0518) -> (-61.2539, 7.7978)
  line L533 (-61.2539, 7.7978) -> (-61.2539, 0.9906)
  line L534 (-61.2539, 0.9906) -> (-62.7459, 0.9906)
  line L535 (-62.7459, 0.9906) -> (-62.7459, 7.7978)
  line L536 (-62.7459, 7.7978) -> (-62.8729, 8.0518)
  line L537 (-62.8729, 8.0518) -> (-63.1269, 8.0518)
  line L538 (-63.1269, 8.0518) -> (-63.2539, 7.7978)
  line L539 (-63.2539, 7.7978) -> (-63.2539, 0.9906)
  line L540 (-63.2539, 0.9906) -> (-64.7459, 0.9906)
  line L541 (-64.7459, 0.9906) -> (-64.7459, 7.7978)
  line L542 (-64.7459, 7.7978) -> (-64.8729, 8.0518)
  line L543 (-64.8729, 8.0518) -> (-65.1269, 8.0518)
  line L544 (-65.1269, 8.0518) -> (-65.2539, 7.7978)
  line L545 (-65.2539, 7.7978) -> (-65.2539, 0.9906)
  line L546 (-65.2539, 0.9906) -> (-66.7459, 0.9906)
  line L547 (-66.7459, 0.9906) -> (-66.7459, 7.7978)
  line L548 (-66.7459, 7.7978) -> (-66.8729, 8.0518)
  line L549 (-66.8729, 8.0518) -> (-67.1269, 8.0518)
  line L550 (-67.1269, 8.0518) -> (-67.2539, 7.7978)
  line L551 (-67.2539, 7.7978) -> (-67.2539, 0.9906)
  line L552 (-67.2539, 0.9906) -> (-68.7459, 0.9906)
  line L553 (-68.7459, 0.9906) -> (-68.7459, 7.7978)
  line L554 (-68.7459, 7.7978) -> (-68.8729, 8.0518)
  line L555 (-68.8729, 8.0518) -> (-69.1269, 8.0518)
  line L556 (-69.1269, 8.0518) -> (-69.2539, 7.7978)
  line L557 (-69.2539, 7.7978) -> (-69.2539, 0.9906)
  line L558 (-69.2539, 0.9906) -> (-70.7459, 0.9906)
  line L559 (-70.7459, 0.9906) -> (-70.7459, 7.7978)
  line L560 (-70.7459, 7.7978) -> (-70.8729, 8.0518)
  line L561 (-70.8729, 8.0518) -> (-71.1269, 8.0518)
  line L562 (-71.1269, 8.0518) -> (-71.2539, 7.7978)
  line L563 (-71.2539, 7.7978) -> (-71.2539, 0.9906)
  line L564 (-71.2539, 0.9906) -> (-72.7459, 0.9906)
  line L565 (-72.7459, 0.9906) -> (-72.7459, 7.7978)
  line L566 (-72.7459, 7.7978) -> (-72.8729, 8.0518)
  line L567 (-72.8729, 8.0518) -> (-73.1269, 8.0518)
  line L568 (-73.1269, 8.0518) -> (-73.2539, 7.7978)
  line L569 (-73.2539, 7.7978) -> (-73.2539, 0.9906)
  line L570 (-73.2539, 0.9906) -> (-74.7459, 0.9906)
  line L571 (-74.7459, 0.9906) -> (-74.7459, 7.7978)
  line L572 (-74.7459, 7.7978) -> (-74.8728, 8.0518)
  line L573 (-74.8728, 8.0518) -> (-75.1268, 8.0518)
  line L574 (-75.1268, 8.0518) -> (-75.2539, 7.7978)
  line L575 (-75.2539, 7.7978) -> (-75.2539, 0.9906)
  line L576 (-75.2539, 0.9906) -> (-76.7458, 0.9906)
  line L577 (-76.7458, 0.9906) -> (-76.7458, 7.7978)
  line L578 (-76.7458, 7.7978) -> (-76.8728, 8.0518)
  line L579 (-76.8728, 8.0518) -> (-77.1268, 8.0518)
  line L580 (-77.1268, 8.0518) -> (-77.2538, 7.7978)
  line L581 (-77.2538, 7.7978) -> (-77.2538, 0.9906)
  line L582 (-77.2538, 0.9906) -> (-78.7458, 0.9906)
  line L583 (-78.7458, 0.9906) -> (-78.7458, 7.7978)
  line L584 (-78.7458, 7.7978) -> (-78.8728, 8.0518)
  line L585 (-78.8728, 8.0518) -> (-79.1268, 8.0518)
  line L586 (-79.1268, 8.0518) -> (-79.2538, 7.7978)
  line L587 (-79.2538, 7.7978) -> (-79.2538, 0.9906)
  line L588 (-79.2538, 0.9906) -> (-80.7458, 0.9906)
  line L589 (-80.7458, 0.9906) -> (-80.7458, 7.7978)
  line L590 (-80.7458, 7.7978) -> (-80.8728, 8.0518)
  line L591 (-80.8728, 8.0518) -> (-81.1268, 8.0518)
  line L592 (-81.1268, 8.0518) -> (-81.2538, 7.7978)
  line L593 (-81.2538, 7.7978) -> (-81.2538, 0.9906)
  line L594 (-81.2538, 0.9906) -> (-82.7458, 0.9906)
  line L595 (-82.7458, 0.9906) -> (-82.7458, 7.7978)
  line L596 (-82.7458, 7.7978) -> (-82.8728, 8.0518)
  line L597 (-82.8728, 8.0518) -> (-83.1268, 8.0518)
  line L598 (-83.1268, 8.0518) -> (-83.2538, 7.7978)
  line L599 (-83.2538, 7.7978) -> (-83.2538, 0.9906)
  line L600 (-83.2538, 0.9906) -> (-84.7458, 0.9906)
  line L601 (-84.7458, 0.9906) -> (-84.7458, 7.7978)
  line L602 (-84.7458, 7.7978) -> (-84.8728, 8.0518)
  line L603 (-84.8728, 8.0518) -> (-85.1268, 8.0518)
  line L604 (-85.1268, 8.0518) -> (-85.2538, 7.7978)
  line L605 (-85.2538, 7.7978) -> (-85.2538, 0.9906)
  line L606 (-85.2538, 0.9906) -> (-86.7458, 0.9906)
  line L607 (-86.7458, 0.9906) -> (-86.7458, 7.7978)
  line L608 (-86.7458, 7.7978) -> (-86.8728, 8.0518)
  line L609 (-86.8728, 8.0518) -> (-87.1268, 8.0518)
  line L610 (-87.1268, 8.0518) -> (-87.2538, 7.7978)
  line L611 (-87.2538, 7.7978) -> (-87.2538, 0.9906)
  line L612 (-87.2538, 0.9906) -> (-88.7458, 0.9906)
  line L613 (-88.7458, 0.9906) -> (-88.7458, 7.7978)
  line L614 (-88.7458, 7.7978) -> (-88.8728, 8.0518)
  line L615 (-88.8728, 8.0518) -> (-89.1268, 8.0518)
  line L616 (-89.1268, 8.0518) -> (-89.2538, 7.7978)
  line L617 (-89.2538, 7.7978) -> (-89.2538, 0.9906)
  line L618 (-89.2538, 0.9906) -> (-90.7458, 0.9906)
  line L619 (-90.7458, 0.9906) -> (-90.7458, 7.7978)
  line L620 (-90.7458, 7.7978) -> (-90.8728, 8.0518)
  line L621 (-90.8728, 8.0518) -> (-91.1268, 8.0518)
  line L622 (-91.1268, 8.0518) -> (-91.2538, 7.7978)
  line L623 (-91.2538, 7.7978) -> (-91.2538, 0.9906)
  line L624 (-91.2538, 0.9906) -> (-92.7458, 0.9906)
  line L625 (-92.7458, 0.9906) -> (-92.7458, 7.7978)
  line L626 (-92.7458, 7.7978) -> (-92.8728, 8.0518)
  line L627 (-92.8728, 8.0518) -> (-93.1268, 8.0518)
  line L628 (-93.1268, 8.0518) -> (-93.2538, 7.7978)
  line L629 (-93.2538, 7.7978) -> (-93.2538, 0.9906)
  line L630 (-93.2538, 0.9906) -> (-93.4603, 0.9906)
  line L631 (-93.4603, 0.9906) -> (-93.4603, 0.762)
  constraints: 1264 end point
extrude "Extrusion2" cut sketch "Sketch_1" along normal mid plane 15.24
ref_plane "0_XY" through (0, 0, 0) normal (0, 1, 0) x (1, 0, 0)
ref_plane "0_YZ" through (0, 0, 0) normal (1, 0, 0) x (0, 0, -1)
ref_plane "0_ZX" through (0, 0, 0) normal (0, 0, -1) x (0, 1, 0)
body "Solid1"
